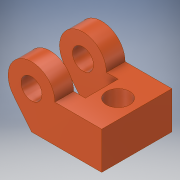
# Autodesk Inventor part: Piston Wall Guide Small
Saved by Autodesk Inventor 2018 (Build 220112000, 112)
## iProperties
Created: 2017-09-27
Part Number: Piston Wall Guide Small
Material: ABS Plastic
Document SubType Name: Modeling
Designer: Gabriel Smolnycki
Density: 1.06 g/cm^3
Appearance: Smooth - Light Orange
Author: Gabriel Smolnycki
Autodesk Inventor part; units mm, degrees
ref_plane "YZ Plane" through (0, 0, 0) normal (1, 0, 0) x (0, 1, 0)
ref_plane "XZ Plane" through (0, 0, 0) normal (0, 1, 0) x (-1, 0, 0)
ref_plane "XY Plane" through (0, 0, 0) normal (0, 0, 1) x (1, 0, 0)
sketch "Sketch1" plane through (0, 0, 0) normal (0, 1, 0) x (-1, 0, 0)
  line L0 (7.5, 7.5) -> (-7.5, 7.5)
  line L1 (-7.5, 7.5) -> (-7.5, -7.5)
  line L2 (-7.5, -7.5) -> (7.5, -7.5)
  line L3 (7.5, -7.5) -> (7.5, 7.5)
  line L4 (7.5, 7.5) -> (-7.5, -7.5) construction
  line L5 (-7.5, 7.5) -> (7.5, -7.5) construction
  point P0 (0, 0)
  dimension "d0" = 15
  dimension "d1" = 15
  constraints: 12 end point, 2 midpoint, 2 parallel, 1 horizontal, 1 perpendicular
  measures "d0" distance of L2.end L1.end
  measures "d1" distance of L1.end L0.end
extrude "Extrusion1" add sketch "Sketch1" along normal blind 8
sketch "Sketch2" plane through (-7.5, 0, 7.5) normal (0, 0, 1) x (1, 0, 0)
  line L0 (0, 8) -> (15, 8) projected
  arc A0 (5, 8) -> (-3.9031, 4.875) centre (0, 8) ccw
  line L1 (0, 0) -> (-3.9031, 4.875)
  line L2 (0, 0) -> (0, 8) projected
  point P0 (7.5, 0)
  dimension "d4" = 10
  constraints: 2 end point, 2 point on circle, 1 centre point, 1 point on line
  measures "d4" diameter of A0
extrude "Extrusion2" add sketch "Sketch2" against normal blind 4
mirror "Mirror1" about plane through (0, 0, 0) normal (0, 0, 1) of "Extrusion2"
sketch "Sketch3" plane through (-7.5, 0, 3.5) normal (0, 0, -1) x (-1, 0, 0)
  arc A0 (3.9031, 4.875) -> (-5, 8) centre (0, 8) ccw projected
  circle A1 centre (0, 8) radius 7.5
  point P0 (-7.5, 0)
  dimension "d7" = 15
  constraints: 1 centre point, 1 coincident
  measures "d7" diameter of A1
extrude "Extrusion3" cut sketch "Sketch3" along normal up to surface (7 mm away)
sketch "Sketch4" plane through (7.5, 0, 7.5) normal (0, 0, 1) x (1, 0, 0)
  arc A0 (-10, 8) -> (-18.9031, 4.875) centre (-15, 8) ccw projected
  point P0 (-7.5, 0)
  constraints: 1 coincident
hole "Hole1" at (-7.5, 8, 7.5) direction (0, 0, -1) diameter 4.5 end through all
sketch "Sketch5" plane through (0, 8, 0) normal (0, 1, 0) x (1, 0, 0)
  line L0 (7.5, -7.5) -> (7.5, 7.5) projected
  point P0 (0, 0)
  point P1 (3.5, 0)
  dimension "d17" = 4
  measures "d17" distance from line of point (3.5, 0) L0
hole "Hole2" at (3.5, 8, 0) direction (0, -1, 0) diameter 5 end through all
body "Solid1"
